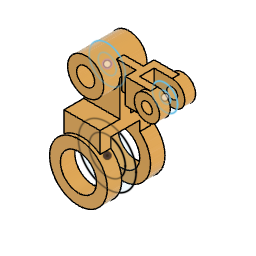
Design 5 v1 (Autodesk Fusion 360 design; units mm, degrees)
Autodesk Fusion 360 part; units mm, degrees
sketch "Sketch1" plane through (0, 0, 0) normal (0, 1, 0) x (1, 0, 0)
  circle A0 centre (0, 0) radius 25
  circle A1 centre (0, 0) radius 40
  circle A2 centre (0, -110) radius 12.5
  circle A3 centre (0, -110) radius 25
  dimension "d1" = 50
  dimension "d2" = 80
  dimension "d3" = 25
  dimension "d4" = 50
  dimension "d5" = 110
  constraint coincident A0.centre A1.centre
  constraint concentric A0 A1
  constraint concentric A2 A3
  measures "d1" diameter of A0
  measures "d2" diameter of A1
  measures "d3" diameter of A2
  measures "d4" diameter of A3
  measures "d5" distance of A0.centre A2.centre
extrude "Extrude1" add sketch "Sketch1" along normal blind 20 from surface at 20 contours A1 makes body 1
sketch "Sketch2" plane through (0, 0, 0) normal (0, 1, 0) x (1, 0, 0)
  circle A0 centre (80, -110) radius 7.5
  circle A1 centre (80, -110) radius 17.5
  point P0 (0, -110)
  dimension "d12" = 15
  dimension "d13" = 35
  dimension "d14" = 80
  constraint concentric A0 A1
  measures "d12" diameter of A0
  measures "d13" diameter of A1
  measures "d14" distance of A0.centre P0
extrude "Extrude2" add sketch "Sketch2" along normal blind 15 from surface at 10 separate body makes body 2
extrude "Extrude3" add sketch "Sketch1" along normal mid plane 60 separate body contours A3 makes body 3
mirror "Mirror1" about plane through (0, 0, 0) normal (0, 1, 0) of bodies 2 1 makes body 4 at (39.9503, -33.3333, 1.9938) makes body 5 at (97.413, -20, 111.7424)
sketch "Sketch3" plane through (0, 0, 0) normal (1, 0, 0) x (0, 1, 0)
  line L0 (35, 0) -> (20, 0)
  line L1 (20, 0) -> (20, 45)
  line L2 (20, 45) -> (35, 45)
  line L3 (35, 45) -> (35, 0)
  line L4 (-20, 0) -> (-35, 0)
  line L5 (-35, 0) -> (-35, 45)
  line L6 (-35, 45) -> (-20, 45)
  line L7 (-20, 45) -> (-20, 0)
  line L8 (-35, 45) -> (35, 45)
  line L9 (35, 45) -> (35, 60)
  line L10 (35, 60) -> (-35, 60)
  line L11 (-35, 60) -> (-35, 45)
  line L12 (-7.5, 45) -> (7.5, 45)
  line L13 (7.5, 45) -> (7.5, 110)
  line L14 (7.5, 110) -> (-7.5, 110)
  line L15 (-7.5, 110) -> (-7.5, 45)
  dimension "d22" = 15
  dimension "d23" = 45
  dimension "d24" = 15
  dimension "d25" = 45
  dimension "d26" = 15
  dimension "d27" = 15
  dimension "d28" = 65
  dimension "d29" = 27.5
  dimension "d30" = 27.5
  constraint horizontal L0
  constraint vertical L1
  constraint horizontal L2
  constraint vertical L3
  constraint horizontal L4
  constraint vertical L5
  constraint horizontal L6
  constraint vertical L7
  constraint horizontal L8
  constraint vertical L9
  constraint horizontal L10
  constraint vertical L11
  constraint horizontal L12
  constraint vertical L13
  constraint horizontal L14
  constraint vertical L15
  constraint coincident L8 L12.start
  constraint collinear L3 L9
  measures "d22" distance of L0.start L0.end
  measures "d23" distance of L0.start L2.end
  measures "d24" distance of L4.start L4.end
  measures "d25" distance of L4.start L6.end
  measures "d26" distance of L5.end L10.end
  measures "d27" distance of L12.start L12.end
  measures "d28" distance of L12.start L14.end
  measures "d29" distance of L9 L13
  measures "d30" distance of L11 L15
extrude "Extrude4" add sketch "Sketch3" along normal mid plane 50 separate body makes body 6
extrude "Extrude5" cut sketch "Sketch1" along normal mid plane 160 contours A0 | A2 bodies 6
ref_plane "WorkPlane1" through (80, 17.5, 110) normal (0, 0, -1) x (0, 1, 0)
sketch "Sketch4" plane through (80, 17.5, 110) normal (0, 0, -1) x (1, 0, 0)
  line L0 (-17.5, 42.5) -> (17.5, 42.5)
  line L1 (-17.5, 27.5) -> (17.5, 27.5)
  line L2 (-17.5, 42.5) -> (-17.5, 27.5)
  line L3 (17.5, 42.5) -> (17.5, 27.5)
  line L4 (-17.5, -7.5) -> (17.5, -7.5)
  line L5 (-17.5, 7.5) -> (17.5, 7.5)
  line L6 (-17.5, 7.5) -> (-17.5, -7.5)
  line L7 (17.5, 7.5) -> (17.5, -7.5)
  line L8 (-55, 47.5) -> (-105, 47.5)
  line L9 (-105, -12.5) -> (-55, -12.5)
  line L10 (-105, 47.5) -> (-105, -12.5)
  line L11 (-55, 47.5) -> (-55, -12.5)
  line L12 (0, 7.5) -> (-25, 7.5)
  line L13 (-25, 7.5) -> (-25, -2.5)
  line L14 (-25, -2.5) -> (0, -2.5)
  line L15 (0, -2.5) -> (0, 7.5)
  line L16 (0, 27.5) -> (-25, 27.5)
  line L17 (-25, 27.5) -> (-25, 37.5)
  line L18 (-25, 37.5) -> (0, 37.5)
  line L19 (0, 37.5) -> (0, 27.5)
  line L20 (-25, 37.5) -> (-35, 37.5)
  line L21 (-35, 37.5) -> (-35, -2.5)
  line L22 (-35, -2.5) -> (-25, -2.5)
  line L23 (-25, -2.5) -> (-25, 37.5)
  line L24 (-25, 22.5) -> (-80, 22.5)
  line L25 (-80, 22.5) -> (-80, 12.5)
  line L26 (-80, 12.5) -> (-25, 12.5)
  line L27 (-25, 12.5) -> (-25, 22.5)
  dimension "d36" = 25
  dimension "d37" = 10
  dimension "d38" = 25
  dimension "d39" = 10
  dimension "d40" = 40
  dimension "d41" = 55
  dimension "d42" = 10
  dimension "d43" = 15
  dimension "d44" = 15
  constraint horizontal L12
  constraint vertical L13
  constraint horizontal L14
  constraint vertical L15
  constraint midpoint L5 L12.start
  constraint horizontal L16
  constraint vertical L17
  constraint horizontal L18
  constraint vertical L19
  constraint midpoint L1 L16.start
  constraint horizontal L20
  constraint vertical L21
  constraint horizontal L22
  constraint vertical L23
  constraint horizontal L24
  constraint vertical L25
  constraint horizontal L26
  constraint vertical L27
  constraint coincident L23 L24.start
  measures "d36" distance of L12.start L12.end
  measures "d37" distance of L12.start L14.end
  measures "d38" distance of L16.start L16.end
  measures "d39" distance of L16.start L18.end
  measures "d40" distance of L17.end L13.end
  measures "d41" distance of L24.start L24.end
  measures "d42" distance of L24.start L26.end
  measures "d43" distance of L22 L26
  measures "d44" distance of L20 L24
extrude "Extrude6" add sketch "Sketch4" along normal mid plane 35 separate body contours L1 L2 L16 L18 L19 | L2 L16 L17 L18 L23 | L17 L20 L21 L23 L24 | L21 L23 L24 L26 L27 | L11 L21 L24 L26 | L13 L21 L22 L23 L26 | L11 L24 L25 L26 | L6 L12 L13 L14 L23 | L5 L6 L12 L14 L15 makes body 7
extrude "Extrude7" cut sketch "Sketch1" sketch "Sketch2" along normal blind 225 contours A2 of sketch 2 contours A0 bodies 7
extrude "Extrude8" cut sketch "Sketch1" along normal mid plane 390 contours A2 bodies 7
extrude "Extrude9" cut sketch "Sketch2" along normal mid plane 100 contours A0 bodies 7
combine "Combine1" operation add target body 6 tool bodies 5 3 2 1 7 4
